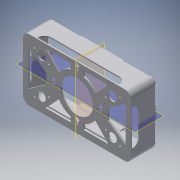
# Autodesk Inventor part: Hub Enclosure Back
Saved by Autodesk Inventor 2018 (Build 220112000, 112)
## iProperties
Created: 2018-03-25
Part Number: Hub Enclosure Back
Material: Generic
Document SubType Name: Modeling
Designer: brutu
Density: 1 g/cm^3
Appearance: White
Author: brutu
Autodesk Inventor part; units mm, degrees
ref_plane "YZ Plane" through (0, 0, 0) normal (1, 0, 0) x (0, 1, 0)
ref_plane "XZ Plane" through (0, 0, 0) normal (0, 1, 0) x (-1, 0, 0)
ref_plane "XY Plane" through (0, 0, 0) normal (0, 0, 1) x (1, 0, 0)
sketch "Sketch1" plane through (0, 0, 0) normal (0, 0, 1) x (1, 0, 0)
  line L0 (77.4925, -45.061) -> (77.4925, 41.939) projected
  line L1 (77.4925, 41.939) -> (-77.5075, 41.939) projected
  line L2 (-77.5075, 41.939) -> (-77.5075, -45.061) projected
  line L3 (-77.5075, -45.061) -> (77.4925, -45.061) projected
  line L4 (85.4725, -56.941) -> (-85.4875, -56.941) projected
  arc A0 (-96.4875, -45.941) -> (-85.4875, -56.941) centre (-85.4875, -45.941) ccw projected
  line L5 (-96.4875, -45.941) -> (-96.4875, 42.819) projected
  arc A1 (-85.4875, 53.819) -> (-96.4875, 42.819) centre (-85.4875, 42.819) ccw projected
  line L6 (-85.4875, 53.819) -> (85.4725, 53.819) projected
  arc A2 (96.4725, 42.819) -> (85.4725, 53.819) centre (85.4725, 42.819) ccw projected
  line L7 (96.4725, 42.819) -> (96.4725, -45.941) projected
  arc A3 (85.4725, -56.941) -> (96.4725, -45.941) centre (85.4725, -45.941) ccw projected
  line L8 (-85.4875, -54.841) -> (85.4725, -54.841)
  arc A4 (85.4725, -54.841) -> (94.3725, -45.941) centre (85.4725, -45.941) ccw
  line L9 (94.3725, -45.941) -> (94.3725, 42.819)
  arc A5 (94.3725, 42.819) -> (85.4725, 51.719) centre (85.4725, 42.819) ccw
  line L10 (85.4725, 51.719) -> (-85.4875, 51.719)
  arc A6 (-85.4875, 51.719) -> (-94.3875, 42.819) centre (-85.4875, 42.819) ccw
  line L11 (-94.3875, 42.819) -> (-94.3875, -45.941)
  arc A7 (-94.3875, -45.941) -> (-85.4875, -54.841) centre (-85.4875, -45.941) ccw
  point P0 (0, 0)
  dimension "d210" = 2.1
  constraints: 8 end point, 8 point on circle, 4 centre point, 7 other
  measures "d210" radial gap between concentric circles of A0 A7
extrude "Extrusion1" add sketch "Sketch1" along normal blind 40.64 contours L4 A0 L5 A1 L6 A2 L7 A3
sketch "Sketch4" plane through (0, 0, 40.64) normal (0, 0, 1) x (1, 0, 0)
  arc A0 (-94.3875, -45.941) -> (-85.4875, -54.841) centre (-85.4875, -45.941) ccw projected
  line L0 (-85.4875, -54.841) -> (85.4725, -54.841) projected
  arc A1 (85.4725, -54.841) -> (94.3725, -45.941) centre (85.4725, -45.941) ccw projected
  line L1 (94.3725, -45.941) -> (94.3725, 42.819) projected
  arc A2 (94.3725, 42.819) -> (85.4725, 51.719) centre (85.4725, 42.819) ccw projected
  line L2 (85.4725, 51.719) -> (-85.4875, 51.719) projected
  arc A3 (-85.4875, 51.719) -> (-94.3875, 42.819) centre (-85.4875, 42.819) ccw projected
  line L3 (-94.3875, 42.819) -> (-94.3875, -45.941) projected
  line L4 (85.4725, -56.941) -> (-85.4875, -56.941) projected
  arc A4 (-96.4875, -45.941) -> (-85.4875, -56.941) centre (-85.4875, -45.941) ccw projected
  line L5 (-96.4875, -45.941) -> (-96.4875, 42.819) projected
  arc A5 (-85.4875, 53.819) -> (-96.4875, 42.819) centre (-85.4875, 42.819) ccw projected
  line L6 (-85.4875, 53.819) -> (85.4725, 53.819) projected
  arc A6 (96.4725, 42.819) -> (85.4725, 53.819) centre (85.4725, 42.819) ccw projected
  line L7 (96.4725, 42.819) -> (96.4725, -45.941) projected
  arc A7 (85.4725, -56.941) -> (96.4725, -45.941) centre (85.4725, -45.941) ccw projected
extrude "Extrusion12" add sketch "Sketch4" along normal blind 2.1 contours L3 A3 L2 A2 L1 A1 L0 A0 | L4 A4 L5 A5 L6 A6 L7 A7
sketch "Sketch7" plane through (0, 0, 42.74) normal (0, 0, 1) x (1, 0, 0)
  line L0 (-2.0288, 41.656) -> (-2.0288, 44.2698)
  line L1 (2.0288, 41.656) -> (2.0288, 44.2698)
  arc A0 (2.0288, 44.2698) -> (-2.0288, 44.2698) centre (0, 47.4948) ccw
  arc A1 (-2.0288, 41.656) -> (2.0288, 41.656) centre (0, 41.656) ccw
  line L2 (-99.48, 47.38) -> (-99.48, -47.38) projected
  line L3 (88.48, 58.38) -> (-88.48, 58.38) projected
  line L4 (39.6272, 0) -> (39.6272, 2.6138)
  line L5 (43.6848, 0) -> (43.6848, 2.6138)
  arc A2 (43.6848, 2.6138) -> (39.6272, 2.6138) centre (41.656, 5.8388) ccw
  arc A3 (39.6272, 0) -> (43.6848, 0) centre (41.656, 0) ccw
  line L6 (2.0288, -41.656) -> (2.0288, -39.0422)
  arc A4 (2.0288, -39.0422) -> (-2.0288, -39.0422) centre (0, -35.8172) ccw
  line L7 (-2.0288, -41.656) -> (-2.0288, -39.0422)
  arc A5 (-2.0288, -41.656) -> (2.0288, -41.656) centre (0, -41.656) ccw
  line L8 (-43.6848, 0) -> (-43.6848, 2.6138)
  arc A6 (-43.6848, 0) -> (-39.6272, 0) centre (-41.656, 0) ccw
  line L9 (-39.6272, 0) -> (-39.6272, 2.6138)
  arc A7 (-39.6272, 2.6138) -> (-43.6848, 2.6138) centre (-41.656, 5.8388) ccw
  circle A8 centre (50.8, -25.4) radius 1.905
  circle A9 centre (-50.8, -25.4) radius 1.905
  circle A10 centre (50.8, 25.4) radius 1.905
  circle A11 centre (-50.8, 25.4) radius 1.905
  circle A12 centre (76.2, -38.1) radius 1.905
  circle A13 centre (-76.2, -38.1) radius 1.905
  circle A14 centre (76.2, 38.1) radius 1.905
  circle A15 centre (-76.2, 38.1) radius 1.905
  point P0 (0, 0)
  dimension "d103" = 3.81
  dimension "d104" = 2.0288
  dimension "d105" = 5.8388
  dimension "d106" = 41.656
  dimension "d107" = 4.0575
  dimension "d113" = 3.81
  dimension "d114" = 2.0288
  dimension "d115" = 5.8388
  dimension "d116" = 4.0575
  dimension "d117" = 41.656
  dimension "d120" = 83.312
  dimension "d127" = 83.312
  dimension "d134" = 3.81
  dimension "d135" = 50.8
  dimension "d136" = 25.4
  dimension "d139" = 101.6
  dimension "d142" = 50.8
  dimension "d145" = 3.81
  dimension "d146" = 76.2
  dimension "d147" = 38.1
  dimension "d150" = 152.4
  dimension "d153" = 76.2
  constraints: 16 centre point, 16 end point, 16 point on circle, 5 vertical, 3 horizontal, 3 vertical alignment, 2 parallel, 1 horizontal alignment, 32 other
  measures "d103" radius of A0
  measures "d104" radius of A1
  measures "d105" distance of A1.centre A0.centre
  measures "d106" distance of point (0, 0) A1.centre
  measures "d107" distance between parallel lines of L1 L0
  measures "d113" radius of A2
  measures "d114" radius of A3
  measures "d115" distance of A3.centre A2.centre
  measures "d116" distance between parallel lines of L5 L4
  measures "d117" distance of point (0, 0) A3.centre
  measures "d120" distance of L1.start L6.start
  measures "d127" distance of L4.start L8.start
  measures "d134" diameter of A8
  measures "d135" horizontal distance of point (0, 0) A8.centre
  measures "d136" vertical distance of point (0, 0) A8.centre
  measures "d139" distance of A8.centre A9.centre
  measures "d142" distance of A8.centre A10.centre
  measures "d145" diameter of A12
  measures "d146" horizontal distance of point (0, 0) A12.centre
  measures "d147" vertical distance of point (0, 0) A12.centre
  measures "d150" distance of A12.centre A13.centre
  measures "d153" distance of A12.centre A14.centre
extrude "Extrusion14" cut sketch "Sketch7" against normal up to next
sketch "Sketch9" plane through (0, 0, 42.74) normal (0, 0, 1) x (1, 0, 0)
  circle A0 centre (0, 0) radius 28.575
  line L0 (-99.48, 47.38) -> (-99.48, -47.38) projected
  line L1 (88.48, 58.38) -> (-88.48, 58.38) projected
  line L2 (-56.0234, 45.68) -> (-11.5734, 45.68)
  line L3 (-11.5734, 45.68) -> (-11.5734, 36.2997)
  line L4 (-56.0234, 45.68) -> (-32.2542, 20.28)
  arc A1 (-11.5734, 36.2997) -> (-32.2542, 20.28) centre (0, 0) ccw
  line L5 (0, 58.38) -> (0, -58.4027)
  line L6 (99.8357, 0) -> (-99.48, 0)
  line L7 (56.0234, 45.68) -> (11.5734, 45.68)
  line L8 (11.5734, 45.68) -> (11.5734, 36.2997)
  line L9 (56.0234, 45.68) -> (32.2542, 20.28)
  arc A2 (32.2542, 20.28) -> (11.5734, 36.2997) centre (0, 0) ccw
  line L10 (-56.0234, -45.68) -> (-11.5734, -45.68)
  line L11 (-11.5734, -45.68) -> (-11.5734, -36.2997)
  line L12 (-56.0234, -45.68) -> (-32.2542, -20.28)
  arc A3 (-32.2542, -20.28) -> (-11.5734, -36.2997) centre (0, 0) ccw
  line L13 (56.0234, -45.68) -> (11.5734, -45.68)
  line L14 (56.0234, -45.68) -> (32.2542, -20.28)
  arc A4 (11.5734, -36.2997) -> (32.2542, -20.28) centre (0, 0) ccw
  line L15 (11.5734, -45.68) -> (11.5734, -36.2997)
  line L16 (-86.78, 31.75) -> (-55.03, 9.525)
  line L17 (-86.78, 31.75) -> (-86.78, -31.75)
  line L18 (-86.78, -31.75) -> (-55.03, -9.525)
  line L19 (-55.03, 9.525) -> (-55.03, -9.525)
  line L20 (86.78, 31.75) -> (55.03, 9.525)
  line L21 (86.78, 31.75) -> (86.78, -31.75)
  line L22 (86.78, -31.75) -> (55.03, -9.525)
  line L23 (55.03, 9.525) -> (55.03, -9.525)
  circle A5 centre (-63.5, 31.75) radius 7.62
  circle A6 centre (-50.8, 25.4) radius 1.905 projected
  circle A7 centre (-76.2, 38.1) radius 1.905 projected
  circle A8 centre (63.5, 31.75) radius 7.62
  circle A9 centre (-63.5, -31.75) radius 7.62
  circle A10 centre (63.5, -31.75) radius 7.62
  point P0 (-86.78, 0)
  point P1 (-86.78, 0)
  point P2 (-55.03, 0)
  point P3 (0.1779, 0)
  dimension "d158" = 57.15
  dimension "d172" = 38.1
  dimension "d173" = 44.45
  dimension "d174" = 25.4
  dimension "d175" = 12.7
  dimension "d176" = 9.3803
  dimension "d178" = 19.05
  dimension "d179" = 63.5
  dimension "d181" = 31.75
  dimension "d182" = 12.7
  dimension "d185" = 15.24
  dimension "d186" = 12.7
  dimension "d187" = 25.4
  dimension "d188" = 12.7
  dimension "d189" = 6.35
  constraints: 44 end point, 20 symmetric about line, 9 centre point, 8 point on circle, 5 midpoint, 3 horizontal alignment, 3 vertical, 2 horizontal, 1 coincident, 1 concentric, 1 perpendicular, 6 other
  measures "d158" diameter of A0
  measures "d172" radius of A1
  measures "d173" distance from line of L2.start L3
  measures "d174" vertical distance of L2.start L4.end
  measures "d175" distance between parallel lines of L1 L2
  measures "d176" distance of L2.end L3.end
  measures "d178" distance of L16.end L18.end
  measures "d179" distance of L16.start L17.end
  measures "d181" distance between parallel lines of L19 L17
  measures "d182" distance between parallel lines of L0 L17
  measures "d185" diameter of A5
  measures "d186" horizontal distance of A5.centre A7.centre
  measures "d187" horizontal distance of A6.centre A7.centre
  measures "d188" vertical distance of A6.centre A7.centre
  measures "d189" vertical distance of A7.centre A5.centre
extrude "Extrusion16" cut sketch "Sketch9" against normal up to next contours L6 L5 A0 | A0 L5 L6 | L5 L6 A0 | A0 L6 L5 | L2 L3 A1 L4 | L21 L22 L23 L6 | L6 L23 L20 L21 | L19 L18 L17 L6 | L6 L17 L16 L19 | L9 A2 L8 L7 | L12 A3 L11 L10 | L13 L15 A4 L14 | A5 | A8 | A9 | A10
sketch "Sketch10" plane through (0, 0, 40.64) normal (0, 0, -1) x (-1, 0, 0)
  line L0 (-55.03, 9.525) -> (-55.03, -9.525) projected
  line L1 (-55.03, -9.525) -> (-86.78, -31.75) projected
  line L2 (-86.78, -31.75) -> (-86.78, 31.75) projected
  line L3 (-86.78, 31.75) -> (-55.03, 9.525) projected
  line L4 (-56.0234, -45.68) -> (-32.2542, -20.28) projected
  arc A0 (-32.2542, -20.28) -> (-11.5734, -36.2997) centre (0, 0) ccw projected
  line L5 (-11.5734, -36.2997) -> (-11.5734, -45.68) projected
  line L6 (-11.5734, -45.68) -> (-56.0234, -45.68) projected
  line L7 (-11.5734, 45.68) -> (-11.5734, 36.2997) projected
  arc A1 (-11.5734, 36.2997) -> (-32.2542, 20.28) centre (0, 0) ccw projected
  line L8 (-32.2542, 20.28) -> (-56.0234, 45.68) projected
  line L9 (-56.0234, 45.68) -> (-11.5734, 45.68) projected
  circle A2 centre (-63.5, -31.75) radius 7.62 projected
  circle A3 centre (-63.5, 31.75) radius 7.62 projected
  circle A4 centre (63.5, 31.75) radius 7.62 projected
  circle A5 centre (63.5, -31.75) radius 7.62 projected
  line L10 (56.0234, 45.68) -> (32.2542, 20.28) projected
  arc A6 (32.2542, 20.28) -> (11.5734, 36.2997) centre (0, 0) ccw projected
  line L11 (11.5734, 36.2997) -> (11.5734, 45.68) projected
  line L12 (11.5734, 45.68) -> (56.0234, 45.68) projected
  line L13 (11.5734, -45.68) -> (11.5734, -36.2997) projected
  arc A7 (11.5734, -36.2997) -> (32.2542, -20.28) centre (0, 0) ccw projected
  line L14 (32.2542, -20.28) -> (56.0234, -45.68) projected
  line L15 (56.0234, -45.68) -> (11.5734, -45.68) projected
  line L16 (86.78, 31.75) -> (86.78, -31.75) projected
  line L17 (86.78, -31.75) -> (55.03, -9.525) projected
  line L18 (55.03, -9.525) -> (55.03, 9.525) projected
  line L19 (55.03, 9.525) -> (86.78, 31.75) projected
  circle A8 centre (0, 0) radius 28.575 projected
  arc A9 (2.0288, -39.0422) -> (-2.0288, -39.0422) centre (0, -35.8172) ccw projected
  line L20 (2.0288, -39.0422) -> (2.0288, -41.656) projected
  arc A10 (-2.0288, -41.656) -> (2.0288, -41.656) centre (0, -41.656) ccw projected
  line L21 (-2.0288, -41.656) -> (-2.0288, -39.0422) projected
  arc A11 (-2.0288, 41.656) -> (2.0288, 41.656) centre (0, 41.656) ccw projected
  line L22 (-2.0288, 41.656) -> (-2.0288, 44.2698) projected
  arc A12 (2.0288, 44.2698) -> (-2.0288, 44.2698) centre (0, 47.4948) ccw projected
  line L23 (2.0288, 44.2698) -> (2.0288, 41.656) projected
  circle A13 centre (-76.2, 38.1) radius 1.905 projected
  circle A14 centre (-76.2, -38.1) radius 1.905 projected
  circle A15 centre (-50.8, 25.4) radius 1.905 projected
  circle A16 centre (-50.8, -25.4) radius 1.905 projected
  circle A17 centre (50.8, -25.4) radius 1.905 projected
  circle A18 centre (50.8, 25.4) radius 1.905 projected
  circle A19 centre (76.2, -38.1) radius 1.905 projected
  circle A20 centre (76.2, 38.1) radius 1.905 projected
  arc A21 (-43.6848, 0) -> (-39.6272, 0) centre (-41.656, 0) ccw projected
  line L24 (-43.6848, 0) -> (-43.6848, 2.6138) projected
  arc A22 (-39.6272, 2.6138) -> (-43.6848, 2.6138) centre (-41.656, 5.8388) ccw projected
  line L25 (-39.6272, 2.6138) -> (-39.6272, 0) projected
  arc A23 (39.6272, 0) -> (43.6848, 0) centre (41.656, 0) ccw projected
  line L26 (39.6272, 0) -> (39.6272, 2.6138) projected
  arc A24 (43.6848, 2.6138) -> (39.6272, 2.6138) centre (41.656, 5.8388) ccw projected
  line L27 (43.6848, 2.6138) -> (43.6848, 0) projected
  line L28 (52.49, -10.8475) -> (89.32, -36.6285)
  line L29 (89.32, -36.6285) -> (89.32, 36.6285)
  line L30 (89.32, 36.6285) -> (52.49, 10.8475)
  line L31 (52.49, 10.8475) -> (52.49, -10.8475)
  line L32 (61.879, -48.22) -> (31.7468, -16.0204)
  arc A25 (9.0334, -34.3935) -> (31.7468, -16.0204) centre (0, 0) ccw
  line L33 (9.0334, -34.3935) -> (9.0334, -48.22)
  line L34 (9.0334, -48.22) -> (61.879, -48.22)
  arc A26 (-31.7468, -16.0204) -> (-9.0334, -34.3935) centre (0, 0) ccw
  line L35 (-31.7468, -16.0204) -> (-61.879, -48.22)
  line L36 (-61.879, -48.22) -> (-9.0334, -48.22)
  line L37 (-9.0334, -48.22) -> (-9.0334, -34.3935)
  line L38 (-52.49, -10.8475) -> (-52.49, 10.8475)
  line L39 (-52.49, 10.8475) -> (-89.32, 36.6285)
  line L40 (-89.32, 36.6285) -> (-89.32, -36.6285)
  line L41 (-89.32, -36.6285) -> (-52.49, -10.8475)
  line L42 (-61.879, 48.22) -> (-31.7468, 16.0204)
  arc A27 (-9.0334, 34.3935) -> (-31.7468, 16.0204) centre (0, 0) ccw
  line L43 (-9.0334, 34.3935) -> (-9.0334, 48.22)
  line L44 (-9.0334, 48.22) -> (-61.879, 48.22)
  line L45 (31.7468, 16.0204) -> (61.879, 48.22)
  line L46 (61.879, 48.22) -> (9.0334, 48.22)
  line L47 (9.0334, 48.22) -> (9.0334, 34.3935)
  arc A28 (31.7468, 16.0204) -> (9.0334, 34.3935) centre (0, 0) ccw
  dimension "d192" = 2.54
  dimension "d193" = 2.54
  dimension "d194" = 2.54
  dimension "d195" = 2.54
  dimension "d196" = 2.54
  dimension "d197" = 2.54
  constraints: 40 end point, 8 point on circle, 4 centre point, 18 other
  measures "d192" distance between parallel lines of L17 L28
  measures "d193" distance between parallel lines of L14 L32
  measures "d194" radial gap between concentric circles of A0 A26
  measures "d195" distance between parallel lines of L0 L38
  measures "d196" distance between parallel lines of L8 L42
  measures "d197" distance between parallel lines of L10 L45
extrude "Extrusion17" add sketch "Sketch10" along normal blind 0.9 contours L31 L30 L29 L28 | L34 L33 A25 L32 | A26 L37 L36 L35 | L41 L40 L39 L38 | L44 L43 A27 L42 | A28 L47 L46 L45
ref_plane "Work Plane4" through (-0.0075, -45.941, 42.74) normal (1, 0, 0) x (0, 0, -1)
ref_plane "Work Plane5" through (-85.4875, -1.561, 42.74) normal (0, -1, 0) x (1, 0, 0)
sketch "Sketch15" plane through (0, 0, 0) normal (0, 0, -1) x (-1, 0, 0)
  line L0 (-94.3725, -45.941) -> (-94.3725, 42.819) projected
  arc A0 (-94.3725, -45.941) -> (-85.4725, -54.841) centre (-85.4725, -45.941) ccw projected
  line L1 (85.4875, -54.841) -> (-85.4725, -54.841) projected
  line L2 (-94.3725, -45.941) -> (-94.3725, 42.819) projected
  arc A1 (-85.4725, 51.719) -> (-94.3725, 42.819) centre (-85.4725, 42.819) ccw projected
  line L3 (-94.3725, -45.941) -> (-94.3725, 42.819) projected
  line L4 (-85.4725, 51.719) -> (85.4875, 51.719) projected
  line L5 (-85.4725, 51.719) -> (85.4875, 51.719) projected
  line L6 (94.3875, 42.819) -> (94.3875, -45.941) projected
  line L7 (94.3875, 42.819) -> (94.3875, -45.941) projected
  arc A2 (85.4875, -54.841) -> (94.3875, -45.941) centre (85.4875, -45.941) ccw projected
  line L8 (94.3875, 42.819) -> (94.3875, -45.941) projected
  line L9 (85.4875, -54.841) -> (-85.4725, -54.841) projected
  line L10 (-66.4225, -54.841) -> (-64.3905, -54.841)
  line L11 (-94.3725, -35.781) -> (-94.3725, -33.749)
  line L12 (67.9615, -54.841) -> (64.4055, -54.841)
  line L13 (94.3875, -35.781) -> (94.3875, -33.749)
  line L14 (94.3875, 32.659) -> (94.3875, 30.627)
  line L15 (94.3875, -45.941) -> (94.3875, 42.819) projected
  line L16 (66.4375, 51.719) -> (64.4055, 51.719)
  line L17 (85.4875, 51.719) -> (-85.4725, 51.719) projected
  line L18 (-94.3725, 30.627) -> (-94.3725, 32.659)
  line L19 (96.4875, -45.941) -> (96.4875, 42.819) projected
  line L20 (-94.3725, 42.819) -> (-94.3725, -45.941) projected
  line L21 (85.4875, -54.841) -> (-85.4725, -54.841) projected
  line L22 (94.3875, -14.261) -> (92.2875, -14.261)
  line L23 (92.2875, -14.261) -> (92.2875, 11.139)
  line L24 (92.2875, 11.139) -> (94.3875, 11.139)
  line L25 (94.3875, 11.139) -> (94.3875, -14.261)
  line L26 (96.4875, -45.941) -> (96.4875, 42.819) projected
  line L27 (38.1075, -54.841) -> (-38.0925, -54.841)
  line L28 (-38.0925, -54.841) -> (-38.0925, -52.741)
  line L29 (-38.0925, -52.741) -> (38.1075, -52.741)
  line L30 (38.1075, -52.741) -> (38.1075, -54.841)
  line L31 (-94.3725, 30.627) -> (-94.3725, -33.749)
  line L32 (-94.3725, -14.261) -> (-92.2725, -14.261)
  line L33 (-92.2725, -14.261) -> (-92.2725, 11.139)
  line L34 (-92.2725, 11.139) -> (-94.3725, 11.139)
  line L35 (85.4875, 51.719) -> (-85.4725, 51.719)
  line L36 (-38.0925, 51.719) -> (-38.0925, 49.619)
  line L37 (-38.0925, 49.619) -> (38.1075, 49.619)
  line L38 (38.1075, 49.619) -> (38.1075, 51.719)
  line L39 (38.1075, 51.719) -> (-38.0925, 51.719)
  line L40 (-94.3725, -14.261) -> (-94.3725, 11.139)
  arc A3 (85.4875, -52.741) -> (92.2875, -45.941) centre (85.4875, -45.941) ccw
  line L41 (85.4875, -52.741) -> (-85.4725, -52.741)
  line L42 (92.2875, -45.941) -> (94.3875, -45.941)
  line L43 (85.4875, -52.741) -> (85.4875, -54.841)
  arc A4 (85.4875, -54.841) -> (94.3875, -45.941) centre (85.4875, -45.941) ccw
  arc A5 (-92.2725, -45.941) -> (-85.4725, -52.741) centre (-85.4725, -45.941) ccw
  line L44 (-85.4725, -52.741) -> (-85.4725, -54.841)
  line L45 (-92.2725, -45.941) -> (-94.3725, -45.941)
  arc A6 (-94.3725, -45.941) -> (-85.4725, -54.841) centre (-85.4725, -45.941) ccw
  arc A7 (94.3875, 42.819) -> (85.4875, 51.719) centre (85.4875, 42.819) ccw projected
  arc A8 (92.2875, 42.819) -> (85.4875, 49.619) centre (85.4875, 42.819) ccw
  line L46 (92.2875, 42.819) -> (94.3875, 42.819)
  line L47 (85.4875, 49.619) -> (85.4875, 51.719)
  arc A9 (94.3875, 42.819) -> (85.4875, 51.719) centre (85.4875, 42.819) ccw
  arc A10 (94.3875, 42.819) -> (85.4875, 51.719) centre (85.4875, 42.819) ccw projected
  arc A11 (-85.4725, 49.619) -> (-92.2725, 42.819) centre (-85.4725, 42.819) ccw
  line L48 (-85.4725, 49.619) -> (85.4875, 49.619)
  line L49 (-85.4725, 49.619) -> (-85.4725, 51.719)
  line L50 (-92.2725, 42.819) -> (-94.3725, 42.819)
  arc A12 (-85.4725, 51.719) -> (-94.3725, 42.819) centre (-85.4725, 42.819) ccw
  point P0 (0, 0)
  point P1 (-64.3905, 51.719)
  point P2 (92.2875, -1.561)
  point P3 (96.4875, -1.561)
  point P4 (96.4875, -33.749)
  point P5 (96.4875, 30.627)
  point P6 (0.0075, -54.841)
  point P7 (0.0075, -54.841)
  point P8 (-92.2725, -1.561)
  point P9 (-94.3725, -1.561)
  dimension "d255" = 25.4
  dimension "d256" = 2.1
  dimension "d259" = 2.1
  dimension "d260" = 76.2
  dimension "d263" = 25.4
  dimension "d264" = 2.1
  dimension "d265" = 2.1
  dimension "d266" = 2.1
  dimension "d267" = 2.1
  constraints: 70 end point, 16 point on circle, 10 perpendicular, 8 centre point, 6 horizontal, 6 midpoint, 4 concentric, 4 parallel, 4 point on line, 3 collinear, 2 horizontal alignment, 2 vertical, 1 coincident, 2 other
  measures "d255" distance of L22.end L23.end
  measures "d256" distance between parallel lines of L25 L23
  measures "d259" distance of L29.end L27.start
  measures "d260" distance of L28.end L29.end
  measures "d263" distance of L33.start L33.end
  measures "d264" radial gap between concentric circles of A2 A3
  measures "d265" radial gap between concentric circles of A0 A5
  measures "d266" radial gap between concentric circles of A7 A8
  measures "d267" radial gap between concentric circles of A1 A11
extrude "Extrusion23" add sketch "Sketch15" along normal mid plane 8.89 contours L45 A5 L44 A0 | L0 L34 L33 L32 | L29 L30 L1 L28 | A3 L42 A2 L43 | A1 L49 A11 L50 | L4 L38 L37 L36 | L22 L23 L24 L6 | L47 A7 L46 A8
chamfer "Chamfer2" distance 2.1 angle 45 8 edges at (-90.2958, 47.6273, 4.445) (-0.0075, 49.619, 4.445) (-92.2875, -1.561, 4.445) (90.2808, 47.6273, 4.445) (94.3725, -1.561, 4.445) (90.2808, -50.7493, 4.445) (-0.0075, -52.741, 4.445) (-90.2958, -50.7493, 4.445)
chamfer "Chamfer3" distance 0.9 angle 45 8 edges at (-0.0075, -54.841, -4.445) (-94.3875, -1.561, -4.445) (-91.7808, -52.2343, -4.445) (-91.7808, 49.1123, -4.445) (-0.0075, 51.719, -4.445) (94.3725, -1.561, -4.445) (91.7658, 49.1123, -4.445) (91.7658, -52.2343, -4.445)
sketch "Sketch16" plane through (-85.4875, 53.819, 42.74) normal (0, 1, 0) x (1, 0, 0)
  line L0 (0, 42.74) -> (170.96, 42.74) projected
  line L1 (0, 42.74) -> (0, 0) projected
  line L2 (170.96, 0) -> (0, 0) projected
  line L3 (170.96, 42.74) -> (170.96, 0) projected
  line L4 (158.26, 0) -> (158.26, 0)
  line L5 (12.7, 0) -> (12.7, 0)
  line L6 (0, 2.1) -> (170.96, 2.1) projected
  line L7 (12.7, 2.1) -> (158.26, 2.1)
  line L8 (158.26, 2.1) -> (158.26, 2.1)
  line L9 (145.56, 14.8) -> (25.4, 14.8)
  line L10 (12.7, 2.1) -> (12.7, 2.1)
  arc A0 (158.26, 2.1) -> (145.56, 14.8) centre (145.56, 2.1) ccw
  arc A1 (25.4, 14.8) -> (12.7, 2.1) centre (25.4, 2.1) ccw
  point P0 (85.4875, 42.74)
  point P1 (12.7, 12.7)
  point P2 (85.48, 0)
  point P3 (85.48, 0)
  point P4 (158.26, 14.8)
  point P5 (85.48, 2.1)
  point P6 (85.48, 2.1)
  dimension "d277" = 12.7
  dimension "d281" = 12.7
  dimension "d282" = 12.7
  dimension "d283" = 12.7
  constraints: 12 end point, 5 point on line, 4 point on circle, 4 tangent, 3 midpoint, 3 parallel, 2 centre point, 2 coincident, 1 equal radius, 1 horizontal, 1 perpendicular
  measures "d277" distance between parallel lines of L1 L5
  measures "d281" distance between parallel lines of L8 L3
  measures "d282" distance of L7.end point (158.26, 14.8)
  measures "d283" radius of A0
extrude "Extrusion24" cut sketch "Sketch16" against normal up to surface (2.1 mm away) contours A1 L9 A0 L6
mirror "Mirror3" about plane through (-85.4875, -1.561, 42.74) normal (0, -1, 0) of "Extrusion24"
sketch "Sketch17" plane through (96.4725, -45.941, 42.74) normal (1, 0, 0) x (0, 0, -1)
  line L0 (42.74, 88.76) -> (42.74, 0) projected
  line L1 (42.74, 88.76) -> (0, 88.76) projected
  line L2 (0, 0) -> (0, 88.76) projected
  line L3 (42.74, 0) -> (0, 0) projected
  line L4 (0, 13.2977) -> (0.2456, 13.2977)
  line L5 (0.2456, 69.2478) -> (0, 69.2478)
  line L6 (0, 0) -> (0, 88.76) projected
  line L7 (2.1, 12.7) -> (2.1, 12.7)
  line L8 (14.8, 25.4) -> (14.8, 63.36)
  line L9 (2.1, 76.06) -> (2.1, 76.06)
  line L10 (2.1, 76.06) -> (2.1, 12.7)
  line L11 (2.1, 88.76) -> (2.1, 0) projected
  arc A0 (2.1, 12.7) -> (14.8, 25.4) centre (2.1, 25.4) ccw
  arc A1 (14.8, 63.36) -> (2.1, 76.06) centre (2.1, 63.36) ccw
  point P0 (42.74, 45.941)
  point P1 (14.8, 12.7)
  point P2 (2.1, 44.38)
  point P3 (2.1, 44.38)
  dimension "d289" = 12.7
  dimension "d290" = 12.7
  dimension "d291" = 12.7
  constraints: 12 end point, 4 point on circle, 4 tangent, 3 parallel, 2 centre point, 2 coincident, 2 horizontal, 2 midpoint, 2 point on line, 1 equal radius, 1 perpendicular
  measures "d289" distance of L7.start point (14.8, 12.7)
  measures "d290" distance between parallel lines of L1 L9
  measures "d291" radius of A0
extrude "Extrusion25" cut sketch "Sketch17" against normal up to surface (2.1 mm away) contours A1 L8 A0 L10
mirror "Mirror4" about plane through (-0.0075, -45.941, 42.74) normal (1, 0, 0) of "Extrusion25"
equation "\"d98\" = d0"
equation "\"d105\" = d103 + d104"
equation "\"d107\" = 2 * d104"
equation "\"d115\" = d113 + d114"
equation "\"d116\" = 2 * d114"
equation "\"d117\" = d106"
equation "\"d120\" = 2 * d117"
equation "\"d127\" = 2 * d117"
equation "\"d139\" = 2 * d135"
equation "\"d142\" = 2 * d136"
equation "\"d150\" = 2 * d146"
equation "\"d153\" = 2 * d147"
equation "\"d186\" = 0.5 * d187"
equation "\"d189\" = 0.5 * d188"
equation "\"d0\" = 2.1"
body "Solid1"
